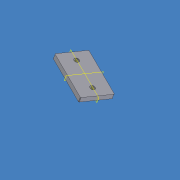
# Autodesk Inventor part: draadlat poot
Saved by Autodesk Inventor 2015 (Build 190159000, 159)
## iProperties
Created: 2007-07-03
Part Number: draadlat poot
Material: Steel, Mild
Document SubType Name: Sheet Metal
Designer: kurt
Manufacturer: Standard
Standards Organization: Custom
Density: 1 g/cm^3
Sheet Metal Rule: Default
Appearance: Steel
Author: kurt
Autodesk Inventor part; units mm, degrees
ref_plane "YZ Plane" through (0, 0, 0) normal (1, 0, 0) x (0, 1, 0)
ref_plane "XZ Plane" through (0, 0, 0) normal (0, 1, 0) x (-1, 0, 0)
ref_plane "XY Plane" through (0, 0, 0) normal (0, 0, 1) x (1, 0, 0)
sketch "Sketch1" plane through (0, 0, 0) normal (0, 0, 1) x (1, 0, 0)
  line L0 (-25, 0) -> (25, 0)
  line L1 (25, 0) -> (25, 80)
  line L2 (25, 80) -> (-25, 80)
  line L3 (-25, 80) -> (-25, 0)
  point P0 (0, 0)
  point P1 (0, 0)
  dimension "d2" = 80
  dimension "d3" = 50
  measures "d2" distance of L0.end L1.end
  measures "d3" distance of L0.start L0.end
extrude "Plate1" add sketch "Sketch1" along normal blind 8
hole "Hole1" at (0, 65, 8) direction (0, 0, -1) diameter 8.376 depth 8 tip angle 118 thread size "M10x1.5" class "6H" standard "ISO Metric profile"
ref_plane "Work Plane1" through (0, 0, 8) normal (-1, 0, 0) x (0, 0, 1)
ref_plane "Work Plane2" through (-25, 40, 8) normal (0, -1, 0) x (1, 0, 0)
mirror "Mirror1" about plane through (-25, 40, 8) normal (0, -1, 0) of "Hole1"
fillet "Corner Round1" radius 1 4 edges at (-25, 0, 4) (25, 0, 4) (-25, 80, 4) (25, 80, 4)
equation "\"d12\" = Thickness"
equation "\"BendReliefWidth\" = Thickness"
equation "\"CornerReliefSize\" = 4 * Thickness"
equation "\"MinimumRemnant\" = 2 * Thickness"
equation "\"TransitionRadius\" = BendRadius"
equation "\"d4\" = BendRadius"
equation "\"JacobiRadiusSize\" = Thickness"
equation "\"GapSize\" = Thickness"
equation "\"Thickness\" = 8"
equation "\"BendRadius\" = 0.001"
body "Solid1"
